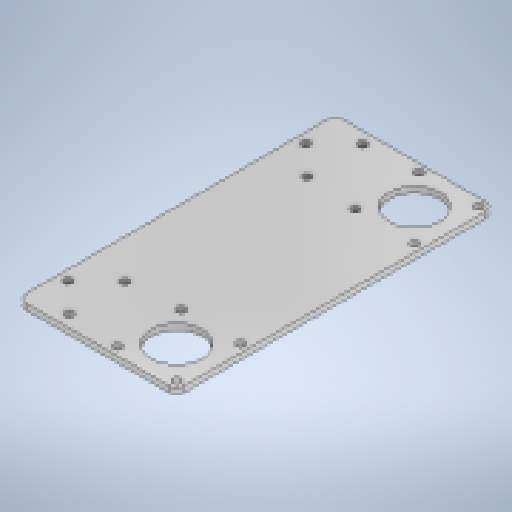
# Autodesk Inventor part: body_bottom_frame
Saved by Autodesk Inventor 2025.2 (Build 292293000, 293)
## iProperties
Created: 2025-08-01
Part Number: body_bottom_frame
Material: Aluminum 6061-AHC
Document SubType Name: Sheet Metal
Designer: chris
Density: 2.7 g/cm^3
Sheet Metal Rule: Default_mm
Appearance: Aluminum - Dark
Author: chris
Autodesk Inventor part; units mm, degrees
ref_plane "YZ Plane" through (0, 0, 0) normal (1, 0, 0) x (0, 1, 0)
ref_plane "XZ Plane" through (0, 0, 0) normal (0, 1, 0) x (-1, 0, 0)
ref_plane "XY Plane" through (0, 0, 0) normal (0, 0, 1) x (1, 0, 0)
sketch "Sketch1" plane through (0, 0, 0) normal (0, 1, 0) x (-1, 0, 0)
  line L0 (-20, 40) -> (20, 40)
  line L1 (20, 40) -> (20, -40)
  line L2 (20, -40) -> (-20, -40)
  line L3 (-20, -40) -> (-20, 40)
  line L4 (-20, 40) -> (20, -40) construction
  line L5 (20, 40) -> (-20, -40) construction
  point P0 (0, 0)
  dimension "d0" = 40
  dimension "d1" = 80
  measures "d0" distance of L1.end L2.end
  measures "d1" distance of L0.end L1.end
extrude "Plate1" add sketch "Sketch1" along normal blind 1.5
fillet "Fillet1" radius 2 4 edges at (20, 0.75, 40) (20, 0.75, -40) (-20, 0.75, -40) (-20, 0.75, 40)
sketch "Sketch2" plane through (0, 0, 0) normal (0, -1, 0) x (1, 0, 0)
  circle A0 centre (-17.42, -29.93) radius 0.7835 projected
  circle A1 centre (-10.12, -22.93) radius 0.7835 projected
  circle A2 centre (-10.12, -36.93) radius 0.7835 projected
  circle A3 centre (3.1, -21.93) radius 0.7835 projected
  circle A4 centre (3.1, -37.93) radius 0.7835 projected
  line L0 (-18.82, -36) -> (-18.82, -23.86) projected
  line L1 (-18.82, -36) -> (-18.1, -36) projected
  arc A5 (-16.1, -38) -> (-18.1, -36) centre (-18.1, -38) ccw projected
  line L2 (-16.1, -38) -> (-16.1, -38.72) projected
  line L3 (16, -38.72) -> (-16.1, -38.72) projected
  line L4 (16, -38.72) -> (16, -38) projected
  arc A6 (18, -36) -> (16, -38) centre (18, -38) ccw projected
  line L5 (18, -36) -> (18.72, -36) projected
  line L6 (18.72, -23.86) -> (18.72, -36) projected
  line L7 (18.72, -23.86) -> (18, -23.86) projected
  arc A7 (16, -21.86) -> (18, -23.86) centre (18, -21.86) ccw projected
  line L8 (16, -21.86) -> (16, -21.14) projected
  line L9 (-16.1, -21.14) -> (16, -21.14) projected
  line L10 (-16.1, -21.14) -> (-16.1, -21.86) projected
  arc A8 (-18.1, -23.86) -> (-16.1, -21.86) centre (-18.1, -21.86) ccw projected
  line L11 (-18.1, -23.86) -> (-18.82, -23.86) projected
  circle A9 centre (10, -29.93) radius 6.4 projected
  circle A10 centre (-17.42, 29.93) radius 0.7835 projected
  circle A11 centre (-10.12, 36.93) radius 0.7835 projected
  circle A12 centre (-10.12, 22.93) radius 0.7835 projected
  circle A13 centre (3.1, 37.93) radius 0.7835 projected
  circle A14 centre (3.1, 21.93) radius 0.7835 projected
  line L12 (-18.82, 23.86) -> (-18.82, 36) projected
  line L13 (-18.82, 23.86) -> (-18.1, 23.86) projected
  arc A15 (-16.1, 21.86) -> (-18.1, 23.86) centre (-18.1, 21.86) ccw projected
  line L14 (-16.1, 21.86) -> (-16.1, 21.14) projected
  line L15 (16, 21.14) -> (-16.1, 21.14) projected
  line L16 (16, 21.14) -> (16, 21.86) projected
  arc A16 (18, 23.86) -> (16, 21.86) centre (18, 21.86) ccw projected
  line L17 (18, 23.86) -> (18.72, 23.86) projected
  line L18 (18.72, 36) -> (18.72, 23.86) projected
  line L19 (18.72, 36) -> (18, 36) projected
  arc A17 (16, 38) -> (18, 36) centre (18, 38) ccw projected
  line L20 (16, 38) -> (16, 38.72) projected
  line L21 (-16.1, 38.72) -> (16, 38.72) projected
  line L22 (-16.1, 38.72) -> (-16.1, 38) projected
  arc A18 (-18.1, 36) -> (-16.1, 38) centre (-18.1, 38) ccw projected
  line L23 (-18.1, 36) -> (-18.82, 36) projected
  circle A19 centre (10, 29.93) radius 6.4 projected
  circle A20 centre (18, 21.86) radius 1 projected
  circle A21 centre (18, 38) radius 1 projected
  circle A22 centre (-18.1, 21.86) radius 1 projected
  circle A23 centre (-18.1, 38) radius 1 projected
  circle A24 centre (-17.42, 29.93) radius 0.7835 projected
  circle A25 centre (-10.12, 36.93) radius 0.7835 projected
  circle A26 centre (-10.12, 22.93) radius 0.7835 projected
  circle A27 centre (3.1, 37.93) radius 0.7835 projected
  circle A28 centre (3.1, 21.93) radius 0.7835 projected
  line L24 (-18.82, 23.86) -> (-18.82, 36) projected
  line L25 (-18.82, 23.86) -> (-18.1, 23.86) projected
  arc A29 (-16.1, 21.86) -> (-18.1, 23.86) centre (-18.1, 21.86) ccw projected
  line L26 (-16.1, 21.86) -> (-16.1, 21.14) projected
  line L27 (16, 21.14) -> (-16.1, 21.14) projected
  line L28 (16, 21.14) -> (16, 21.86) projected
  arc A30 (18, 23.86) -> (16, 21.86) centre (18, 21.86) ccw projected
  line L29 (18, 23.86) -> (18.72, 23.86) projected
  line L30 (18.72, 36) -> (18.72, 23.86) projected
  line L31 (18.72, 36) -> (18, 36) projected
  arc A31 (16, 38) -> (18, 36) centre (18, 38) ccw projected
  line L32 (16, 38) -> (16, 38.72) projected
  line L33 (-16.1, 38.72) -> (16, 38.72) projected
  line L34 (-16.1, 38.72) -> (-16.1, 38) projected
  arc A32 (-18.1, 36) -> (-16.1, 38) centre (-18.1, 38) ccw projected
  line L35 (-18.1, 36) -> (-18.82, 36) projected
  circle A33 centre (10, 29.93) radius 6.4 projected
  circle A34 centre (-17.42, -29.93) radius 0.7835 projected
  circle A35 centre (-10.12, -22.93) radius 0.7835 projected
  circle A36 centre (-10.12, -36.93) radius 0.7835 projected
  circle A37 centre (3.1, -21.93) radius 0.7835 projected
  circle A38 centre (3.1, -37.93) radius 0.7835 projected
  line L36 (-18.82, -36) -> (-18.82, -23.86) projected
  line L37 (-18.82, -36) -> (-18.1, -36) projected
  arc A39 (-16.1, -38) -> (-18.1, -36) centre (-18.1, -38) ccw projected
  line L38 (-16.1, -38) -> (-16.1, -38.72) projected
  line L39 (16, -38.72) -> (-16.1, -38.72) projected
  line L40 (16, -38.72) -> (16, -38) projected
  arc A40 (18, -36) -> (16, -38) centre (18, -38) ccw projected
  line L41 (18, -36) -> (18.72, -36) projected
  line L42 (18.72, -23.86) -> (18.72, -36) projected
  line L43 (18.72, -23.86) -> (18, -23.86) projected
  arc A41 (16, -21.86) -> (18, -23.86) centre (18, -21.86) ccw projected
  line L44 (16, -21.86) -> (16, -21.14) projected
  line L45 (-16.1, -21.14) -> (16, -21.14) projected
  line L46 (-16.1, -21.14) -> (-16.1, -21.86) projected
  arc A42 (-18.1, -23.86) -> (-16.1, -21.86) centre (-18.1, -21.86) ccw projected
  line L47 (-18.1, -23.86) -> (-18.82, -23.86) projected
  circle A43 centre (10, -29.93) radius 6.4 projected
  circle A44 centre (18, -21.86) radius 1 projected
  circle A45 centre (18, -38) radius 1 projected
  circle A46 centre (-18.1, -38) radius 1 projected
  circle A47 centre (-18.1, -21.86) radius 1 projected
  point P0 (0, 0)
hole "Hole1" at (-17.42, 0, 29.93) at (-10.12, 0, 22.93) at (-10.12, 0, 36.93) at (3.1, 0, 37.93) at (3.1, 0, 21.93) at (3.1, 0, -21.93) at (3.1, 0, -37.93) at (-10.12, 0, -22.93) at (-17.42, 0, -29.93) at (-10.12, 0, -36.93) direction (0, 1, 0) diameter 2.1 end through all
sketch "Sketch3" plane through (0, 0, 0) normal (0, -1, 0) x (1, 0, 0)
  circle A0 centre (-17.42, 29.93) radius 0.7835 projected
  circle A1 centre (-10.12, 36.93) radius 0.7835 projected
  circle A2 centre (-10.12, 22.93) radius 0.7835 projected
  circle A3 centre (3.1, 37.93) radius 0.7835 projected
  circle A4 centre (3.1, 21.93) radius 0.7835 projected
  line L0 (-18.82, 23.86) -> (-18.82, 36) projected
  line L1 (-18.82, 23.86) -> (-18.1, 23.86) projected
  arc A5 (-16.1, 21.86) -> (-18.1, 23.86) centre (-18.1, 21.86) ccw projected
  line L2 (-16.1, 21.86) -> (-16.1, 21.14) projected
  line L3 (16, 21.14) -> (-16.1, 21.14) projected
  line L4 (16, 21.14) -> (16, 21.86) projected
  arc A6 (18, 23.86) -> (16, 21.86) centre (18, 21.86) ccw projected
  line L5 (18, 23.86) -> (18.72, 23.86) projected
  line L6 (18.72, 36) -> (18.72, 23.86) projected
  line L7 (18.72, 36) -> (18, 36) projected
  arc A7 (16, 38) -> (18, 36) centre (18, 38) ccw projected
  line L8 (16, 38) -> (16, 38.72) projected
  line L9 (-16.1, 38.72) -> (16, 38.72) projected
  line L10 (-16.1, 38.72) -> (-16.1, 38) projected
  arc A8 (-18.1, 36) -> (-16.1, 38) centre (-18.1, 38) ccw projected
  line L11 (-18.1, 36) -> (-18.82, 36) projected
  circle A9 centre (10, 29.93) radius 6.4 projected
  circle A10 centre (-17.42, -29.93) radius 0.7835 projected
  circle A11 centre (-10.12, -22.93) radius 0.7835 projected
  circle A12 centre (-10.12, -36.93) radius 0.7835 projected
  circle A13 centre (3.1, -21.93) radius 0.7835 projected
  circle A14 centre (3.1, -37.93) radius 0.7835 projected
  line L12 (-18.82, -36) -> (-18.82, -23.86) projected
  line L13 (-18.82, -36) -> (-18.1, -36) projected
  arc A15 (-16.1, -38) -> (-18.1, -36) centre (-18.1, -38) ccw projected
  line L14 (-16.1, -38) -> (-16.1, -38.72) projected
  line L15 (16, -38.72) -> (-16.1, -38.72) projected
  line L16 (16, -38.72) -> (16, -38) projected
  arc A16 (18, -36) -> (16, -38) centre (18, -38) ccw projected
  line L17 (18, -36) -> (18.72, -36) projected
  line L18 (18.72, -23.86) -> (18.72, -36) projected
  line L19 (18.72, -23.86) -> (18, -23.86) projected
  arc A17 (16, -21.86) -> (18, -23.86) centre (18, -21.86) ccw projected
  line L20 (16, -21.86) -> (16, -21.14) projected
  line L21 (-16.1, -21.14) -> (16, -21.14) projected
  line L22 (-16.1, -21.14) -> (-16.1, -21.86) projected
  arc A18 (-18.1, -23.86) -> (-16.1, -21.86) centre (-18.1, -21.86) ccw projected
  line L23 (-18.1, -23.86) -> (-18.82, -23.86) projected
  circle A19 centre (10, -29.93) radius 6.4 projected
  point P0 (0, 0)
extrude "Cut1" cut sketch "Sketch3" against normal blind 1.5 contours A9 | A19
sketch "Sketch4" plane through (0, 0, 0) normal (0, -1, 0) x (1, 0, 0)
  circle A0 centre (-17.42, 29.93) radius 0.7835 projected
  circle A1 centre (-10.12, 36.93) radius 0.7835 projected
  circle A2 centre (-10.12, 22.93) radius 0.7835 projected
  circle A3 centre (3.1, 37.93) radius 0.7835 projected
  circle A4 centre (3.1, 21.93) radius 0.7835 projected
  line L0 (-18.82, 23.86) -> (-18.82, 36) projected
  line L1 (-18.82, 23.86) -> (-18.1, 23.86) projected
  arc A5 (-16.1, 21.86) -> (-18.1, 23.86) centre (-18.1, 21.86) ccw projected
  line L2 (-16.1, 21.86) -> (-16.1, 21.14) projected
  line L3 (16, 21.14) -> (-16.1, 21.14) projected
  line L4 (16, 21.14) -> (16, 21.86) projected
  arc A6 (18, 23.86) -> (16, 21.86) centre (18, 21.86) ccw projected
  line L5 (18, 23.86) -> (18.72, 23.86) projected
  line L6 (18.72, 36) -> (18.72, 23.86) projected
  line L7 (18.72, 36) -> (18, 36) projected
  arc A7 (16, 38) -> (18, 36) centre (18, 38) ccw projected
  line L8 (16, 38) -> (16, 38.72) projected
  line L9 (-16.1, 38.72) -> (16, 38.72) projected
  line L10 (-16.1, 38.72) -> (-16.1, 38) projected
  arc A8 (-18.1, 36) -> (-16.1, 38) centre (-18.1, 38) ccw projected
  line L11 (-18.1, 36) -> (-18.82, 36) projected
  circle A9 centre (10, 29.93) radius 6.4 projected
  circle A10 centre (-17.42, -29.93) radius 0.7835 projected
  circle A11 centre (-10.12, -22.93) radius 0.7835 projected
  circle A12 centre (-10.12, -36.93) radius 0.7835 projected
  circle A13 centre (3.1, -21.93) radius 0.7835 projected
  circle A14 centre (3.1, -37.93) radius 0.7835 projected
  line L12 (-18.82, -36) -> (-18.82, -23.86) projected
  line L13 (-18.82, -36) -> (-18.1, -36) projected
  arc A15 (-16.1, -38) -> (-18.1, -36) centre (-18.1, -38) ccw projected
  line L14 (-16.1, -38) -> (-16.1, -38.72) projected
  line L15 (16, -38.72) -> (-16.1, -38.72) projected
  line L16 (16, -38.72) -> (16, -38) projected
  arc A16 (18, -36) -> (16, -38) centre (18, -38) ccw projected
  line L17 (18, -36) -> (18.72, -36) projected
  line L18 (18.72, -23.86) -> (18.72, -36) projected
  line L19 (18.72, -23.86) -> (18, -23.86) projected
  arc A17 (16, -21.86) -> (18, -23.86) centre (18, -21.86) ccw projected
  line L20 (16, -21.86) -> (16, -21.14) projected
  line L21 (-16.1, -21.14) -> (16, -21.14) projected
  line L22 (-16.1, -21.14) -> (-16.1, -21.86) projected
  arc A18 (-18.1, -23.86) -> (-16.1, -21.86) centre (-18.1, -21.86) ccw projected
  line L23 (-18.1, -23.86) -> (-18.82, -23.86) projected
  circle A19 centre (10, -29.93) radius 6.4 projected
  point P0 (0, 0)
hole "Hole2" at (18, 0, 21.86) at (18, 0, 38) at (18, 0, -21.86) at (18, 0, -38) direction (0, 1, 0) diameter 2.1 end through all
equation "\"d9\" = Thickness"
equation "\"d11\" = Thickness"
equation "\"d18\" = Thickness"
equation "\"d2\" = Thickness"
equation "\"BendReliefWidth\" = Thickness"
equation "\"BendReliefDepth\" = 0.5 * Thickness"
equation "\"CornerReliefSize\" = 4 * Thickness"
equation "\"MinimumRemnant\" = 2 * Thickness"
equation "\"TransitionRadius\" = BendRadius"
equation "\"JacobiRadiusSize\" = BendRadius"
equation "\"GapSize\" = Thickness"
equation "\"Thickness\" = 1.5"
equation "\"BendRadius\" = 0.31"
body "Solid1"
